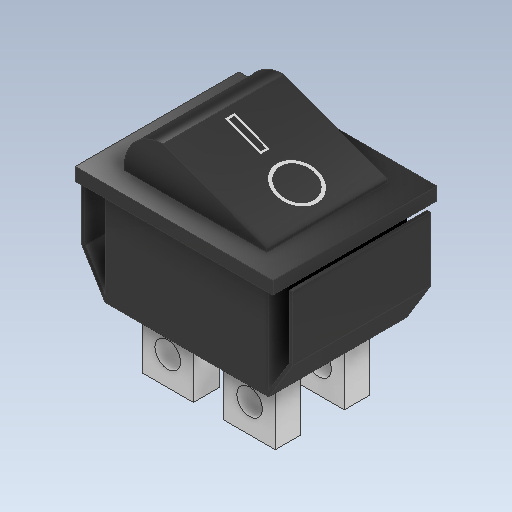
# Autodesk Inventor part: Tecla On_Off - LED
Saved by Autodesk Inventor 2020 (Build 240168000, 168)
## iProperties
Created: 2020-06-18
Part Number: Tecla On_Off - LED
Material: Generic
Document SubType Name: Modeling
Designer: Dante
Density: 1 g/cm^3
Appearance: Default
Author: Dante
Autodesk Inventor part; units mm, degrees
ref_plane "YZ Plane" through (0, 0, 0) normal (1, 0, 0) x (0, 1, 0)
ref_plane "XZ Plane" through (0, 0, 0) normal (0, 1, 0) x (-1, 0, 0)
ref_plane "XY Plane" through (0, 0, 0) normal (0, 0, 1) x (1, 0, 0)
sketch "Sketch1" plane through (0, 0, 0) normal (0, 0, 1) x (1, 0, 0)
  line L0 (0, -2) -> (30.8, -2)
  line L1 (4.3, -2) -> (4.3, -1.5)
  line L2 (30.8, -2) -> (30.8, -4)
  line L3 (30.8, -4) -> (0, -4)
  line L4 (0, -4) -> (0, -2)
  line L5 (2.65, -20) -> (28.15, -20)
  line L6 (2.65, -20) -> (2.65, -4)
  line L7 (28.15, -20) -> (28.15, -4)
  arc A0 (10.3, 4.5) -> (4.3, -1.5) centre (10.3, -1.5) ccw
  line L8 (10.3, 4.5) -> (26.5, -1.5)
  line L9 (26.5, -1.5) -> (26.5, -2)
  line L10 (-1, -14) -> (2.65, -20)
  line L11 (-1, -14) -> (-1, -4)
  line L12 (-0.5, -4) -> (-0.5, -13.8599)
  line L13 (-0.5, -13.8599) -> (2.65, -19.0379)
  line L14 (-1, -4) -> (-0.5, -4)
  line L15 (31.8, -14) -> (28.15, -20)
  line L16 (31.8, -14) -> (31.8, -4)
  line L17 (31.3, -4) -> (31.3, -13.8599)
  line L18 (31.3, -13.8599) -> (28.15, -19.0379)
  line L19 (31.8, -4) -> (31.3, -4)
  point P0 (4.3, 4.5)
  dimension "d0" = 30.8
  dimension "d2" = 6.5
  dimension "d4" = 2
  dimension "d6" = 4.3
  dimension "d9" = 25.5
  dimension "d10" = 16
  dimension "d11" = 6
  dimension "d12" = 0.5
  dimension "d13" = 6
  dimension "d16" = 6
  dimension "d17" = 10
  dimension "d19" = 0.5
  constraints: 40 end point, 6 point on line, 6 vertical, 4 horizontal, 2 perpendicular, 2 point on circle, 1 centre point, 1 tangent
  measures "d0" distance of L0.start L0.end
  measures "d2" distance of L1.start point (4.3, 4.5)
  measures "d4" distance of L0.end L2.end
  measures "d6" distance between parallel lines of L4 L1
  measures "d9" distance of L5.start L5.end
  measures "d10" distance of L5.start L6.end
  measures "d11" radius of A0
  measures "d12" distance of L8.end L9.end
  measures "d13" vertical distance of L8.end L8.start
  measures "d16" vertical distance of L10.start L5.start
  measures "d17" distance of L10.start L11.end
  measures "d19" distance between parallel lines of L11 L12
extrude "Extrusion1" add sketch "Sketch1" along normal blind 25.5 contours L0 L2 L3 L4
extrude "Extrusion2" add sketch "Sketch1" along normal blind 22.15 contours L1 A0 L8 L9 L0
sketch "Sketch2" plane through (30.8, -4, 0) normal (1, 0, 0) x (0, 0, -1)
  line L0 (-3.35, 8.5) -> (-3.35, 2)
  line L1 (0, 8.5) -> (-22.15, 8.5) projected
  line L2 (-3.35, 8.5) -> (0, 8.5)
  line L3 (0, 0) -> (-25.5, 0) projected
  line L4 (0, 2) -> (-22.15, 2) projected
  line L5 (-3.35, 2) -> (0, 2)
  line L6 (0, 2) -> (0, 8.5)
  point P0 (0, 4)
  constraints: 8 end point, 2 collinear, 2 point on line, 1 perpendicular
extrude "Extrusion3" cut sketch "Sketch2" against normal blind 30
extrude "Extrusion4" add sketch "Sketch1" along normal blind 23.5 contours L3 L7 L5 L6 | L6 L10 L11 L14 L12 L13 | L18 L17 L19 L16 L15 L7
sketch "Sketch3" plane through (31.8, -14, 0) normal (1, 0, 0) x (0, 0, -1)
  line L0 (0, 10) -> (-25.5, 10) projected
  line L1 (0, 10) -> (-2, 10)
  line L2 (-2, 10) -> (-2, -9.6179)
  line L3 (-2, -9.6179) -> (0, -9.6179)
  line L4 (0, -5.0379) -> (0, 10) projected
  line L5 (0, -9.6179) -> (0, 10)
  line L6 (0, 10) -> (0, -9.6179)
  point P0 (0, 14)
  dimension "d29" = 2
  constraints: 10 end point, 2 collinear, 2 perpendicular, 1 point on line
  measures "d29" distance of L0.start L1.end
extrude "Extrusion5" cut sketch "Sketch3" against normal blind 40
sketch "Sketch4" plane through (2.65, -20, 23.5) normal (0, -1, 0) x (1, 0, 0)
  line L0 (25.5, -21.5) -> (25.5, 0) projected
  line L1 (25.5, -21.5) -> (0, 0)
  line L2 (12.75, -10.75) -> (12.75, -21.5)
  line L3 (0, -21.5) -> (25.5, -21.5) projected
  line L4 (12.75, -21.5) -> (25.5, -21.5)
  line L5 (19.125, -21.5) -> (19.125, 0)
  line L6 (0, 0) -> (25.5, 0) projected
  line L7 (19.125, -16.125) -> (15.125, -16.125)
  line L8 (15.125, -16.125) -> (15.125, -18.125)
  line L9 (15.125, -18.125) -> (23.125, -18.125)
  line L10 (23.125, -18.125) -> (23.125, -14.125)
  line L11 (23.125, -14.125) -> (15.125, -14.125)
  line L12 (15.125, -14.125) -> (15.125, -16.125)
  line L13 (12.75, -10.75) -> (9.9991, -10.75)
  line L14 (10.375, -16.125) -> (10.375, -18.125)
  line L15 (10.375, -18.125) -> (2.375, -18.125)
  line L16 (2.375, -18.125) -> (2.375, -14.125)
  line L17 (2.375, -14.125) -> (10.375, -14.125)
  line L18 (10.375, -14.125) -> (10.375, -16.125)
  line L19 (15.125, -5.375) -> (15.125, -3.375)
  line L20 (15.125, -3.375) -> (23.125, -3.375)
  line L21 (23.125, -3.375) -> (23.125, -7.375)
  line L22 (23.125, -7.375) -> (15.125, -7.375)
  line L23 (15.125, -7.375) -> (15.125, -5.375)
  line L24 (10.375, -5.375) -> (10.375, -3.375)
  line L25 (10.375, -3.375) -> (2.375, -3.375)
  line L26 (2.375, -3.375) -> (2.375, -7.375)
  line L27 (2.375, -7.375) -> (10.375, -7.375)
  line L28 (10.375, -7.375) -> (10.375, -5.375)
  line L29 (19.125, -14.125) -> (16.7529, -14.125)
  line L30 (19.125, -7.375) -> (15.125, -7.375)
  line L31 (15.125, -3.375) -> (15.125, -7.375)
  line L32 (19.125, -3.375) -> (15.125, -3.375)
  point P0 (-2.65, -23.5)
  dimension "d32" = 4
  dimension "d33" = 2
  dimension "d34" = 8
  dimension "d35" = 4
  constraints: 60 end point, 15 symmetric about line, 9 point on line, 7 perpendicular, 5 midpoint, 3 collinear, 2 horizontal, 1 vertical
  measures "d32" distance of L7.start L7.end
  measures "d33" distance of L7.end L8.end
  measures "d34" distance of L8.end L9.end
  measures "d35" distance of L9.end L10.end
extrude "Extrusion6" add sketch "Sketch4" along normal blind 10 contours L9 L5 L1 | L1 L5 L11 L10 L9 | L7 L12 L11 L1 | L1 L11 L5 | L5 L9 L8 L7 | L20 L21 L22 L5 | L5 L22 L23 L19 L20 | L25 L24 L28 L27 L1 | L1 L27 L26 L25 | L14 L15 L16 L17 L18
sketch "Sketch5" plane through (25.775, -20, 5.375) normal (0, 0, -1) x (-1, 0, 0)
  circle A0 centre (4, -5.5341) radius 2
  line L0 (23.125, 0) -> (-2.375, 0) projected
  line L1 (10.375, 0) -> (10.375, -1.7461)
  circle A1 centre (16.75, -5.5341) radius 2
  dimension "d38" = 4
  constraints: 2 centre point, 2 end point, 1 midpoint, 1 symmetric about line, 1 vertical, 1 other
  measures "d38" diameter of A0
extrude "Extrusion7" cut sketch "Sketch5" against normal blind 40
sketch "Sketch6" plane through (10.3, 4.5, 22.15) normal (0.3473, 0.9377, 0) x (0.9377, -0.3473, 0)
  line L0 (17.2754, 18.8) -> (17.2754, 0) projected
  line L1 (17.2754, 9.4) -> (-10.0504, 9.4)
  line L2 (17.4491, 0) -> (-3.3689, 0) projected
  line L3 (7.0401, 0) -> (7.0357, 14.775)
  line L4 (7.0357, 12.775) -> (7.0357, 16.775) projected
  line L5 (7.0373, 9.4) -> (17.4491, 0)
  circle A0 centre (12.2432, 9.4) radius 2.75
  line L6 (7.0401, 0) -> (0, 9.4)
  line L7 (0, 18.8) -> (0, 0) projected
  line L8 (7.0373, 9.4) -> (7.0375, 8.65)
  line L9 (7.0375, 8.65) -> (1.0375, 8.6482)
  line L10 (1.0375, 8.6482) -> (1.0371, 10.1482)
  line L11 (1.0371, 10.1482) -> (7.0371, 10.15)
  line L12 (7.0373, 9.4) -> (7.0371, 10.15)
  line L13 (1.0371, 10.1482) -> (7.0371, 10.15)
  circle A1 centre (12.2432, 9.4) radius 3.35
  line L14 (1.4371, 10.1484) -> (1.4374, 9.0484)
  line L15 (1.4374, 9.0484) -> (6.6374, 9.0499)
  line L16 (6.6374, 9.0499) -> (6.6373, 9.3999)
  line L17 (1.0372, 9.7482) -> (7.0372, 9.75)
  line L18 (6.6373, 9.3999) -> (6.6371, 10.1499)
  point P0 (-8.0959, 22.15)
  point P1 (1.4372, 9.7484)
  point P2 (6.6372, 9.7499)
  dimension "d41" = 5.5
  dimension "d42" = 0.75
  dimension "d43" = 6
  dimension "d44" = 1.5
  dimension "d45" = 0.6
  dimension "d46" = 0.4
  dimension "d47" = 0.4
  dimension "d48" = 0.4
  constraints: 30 end point, 5 perpendicular, 5 point on line, 4 midpoint, 2 centre point, 2 collinear, 2 parallel, 1 horizontal, 2 other
  measures "d41" diameter of A0
  measures "d42" distance of L5.start L8.end
  measures "d43" distance of L8.end L9.end
  measures "d44" distance of L9.end L10.end
  measures "d45" radial gap between concentric circles of A0 A1
  measures "d46" distance between parallel lines of L9 L15
  measures "d47" distance between parallel lines of L11 L17
  measures "d48" distance between parallel lines of L12 L18
extrude "Extrusion8" add sketch "Sketch6" along normal blind 0.01 contours A1 L1 A0 | L1 A0 A1 | L3 L9 L10 L1 L14 L15 L16 | L1 L18 L17 L3 | L17 L18 L11 L3 | L1 L10 L17 L14 | L17 L14 L11 L18 | L17 L10 L11 L14
sketch "Sketch7" plane through (13.025, -20, 5.375) normal (0, 0, -1) x (-1, 0, 0)
  circle A0 centre (4, -5.5341) radius 2 projected
body "Solid1"
